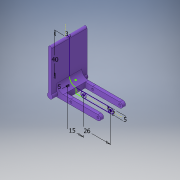
# Autodesk Inventor part: Mouth-Height-Lever-front
Saved by Autodesk Inventor 2018.3 (Build 223284000, 284)
## iProperties
Created: 2018-05-17
Part Number: Mouth-Height-Lever-front
Material: Generisch
Document SubType Name: Modeling
Designer: JochenAlt
Density: 1 g/cm^3
Appearance: Violett
Author: JochenAlt
Autodesk Inventor part; units mm, degrees
ref_plane "YZ Plane" through (0, 0, 0) normal (1, 0, 0) x (0, 1, 0)
ref_plane "XZ Plane" through (0, 0, 0) normal (0, 1, 0) x (-1, 0, 0)
ref_plane "XY Plane" through (0, 0, 0) normal (0, 0, 1) x (1, 0, 0)
sketch "Skizze4" plane through (0, 0, 0) normal (0, 1, 0) x (-1, 0, 0)
  line L0 (-43.5, 2.5) -> (-2.5, 2.5) construction
  line L1 (0, -11.3) -> (0, 50.3) construction
  line L2 (-55.2, 0) -> (9.2, 0) construction
  circle A0 centre (-43.5, 0) radius 2.5
  circle A1 centre (-43.5, 0) radius 1
  circle A2 centre (-2.5, 0) radius 2.5
  line L3 (-12.1436, -2.5) -> (-43.5, -2.5) construction
  circle A3 centre (-17.5, 0) radius 2.5
  line L4 (-43.5, 2.5) -> (-17.5, 2.5)
  line L5 (-43.5, -2.5) -> (-17.5, -2.5)
  line L6 (-1, 2) -> (-1, 40)
  arc A4 (-1, 40) -> (-4, 40) centre (-2.5, 40) ccw
  circle A5 centre (-17.5, 0) radius 1
  line L7 (-4, 8.7208) -> (-4, 40)
  line L8 (-10.2208, 2.5) -> (-2.5, 2.5)
  line L9 (-2.5, 0) -> (-2.5, 40) construction
  line L10 (-4, 8.7208) -> (-4, 2.5)
  arc A6 (-10.2208, 2.5) -> (-4, 8.7208) centre (-10.2208, 8.7208) ccw
  line L11 (-4, 2.5) -> (-4, 2)
  line L12 (-10.2208, 2.5) -> (-10.2208, -2.5)
  line L13 (-10.2208, -2.5) -> (-2.5, -2.5)
  line L14 (-10.2208, 2.5) -> (-17.5, 2.5)
  line L15 (-10.2208, -2.5) -> (-17.5, -2.5)
  arc A7 (-17.5, -2.5) -> (-17.5, 2.5) centre (-17.5, 0) ccw
  point P0 (0, 0)
  point P1 (-2.5, -2.5)
  point P2 (-2.5, -2.5)
  dimension "d35" = 5
  dimension "d28" = 2
  dimension "d30" = 15
  dimension "d32" = 26
  dimension "d33" = 5
  dimension "d41" = 3
  dimension "d43" = 40
  constraints: 28 end point, 12 point on circle, 10 tangent, 7 centre point, 5 horizontal, 4 parallel, 4 vertical, 2 coincident, 2 perpendicular, 1 equal radius, 1 point on line, 10 other
  measures "d28" diameter of A1
  measures "d30" distance of L9.start A3.centre
  measures "d32" distance of A3.centre A0.centre
  measures "d33" distance between parallel lines of L5 L4
  measures "d41" distance between parallel lines of L6 L7
  measures "d43" distance from line of L2 L9.end
extrude "Extrusion6" add sketch "Skizze4" along normal mid plane 24 contours A0 | A0 L4 A3 L5 | L14 L12 L15 A3 | A3 | A6 L10 L8 | L8 L11 A2 L13 L12
extrude "Extrusion8" add sketch "Skizze4" along normal mid plane 34 contours L10 L7 A4 L6 A2 L8 | L8 A2 L11 | A2
extrude "Extrusion7" cut sketch "Skizze4" along normal mid plane 18 contours A0 | A0 L4 A3 L5 | L14 L12 L15 A3 | A3 | A1
